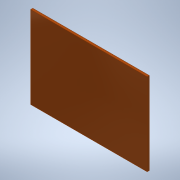
# Autodesk Inventor part: Yplate
Saved by Autodesk Inventor 2020 (Build 240168000, 168)
## iProperties
Created: 2019-06-14
Part Number: Yplate
Material: Phenolic Resin
Document SubType Name: Modeling
Designer: LillaHunden
Density: 1.38 g/cm^3
Appearance: Smooth - Light Orange
Author: LillaHunden
Autodesk Inventor part; units mm, degrees
ref_plane "YZ Plane" through (0, 0, 0) normal (1, 0, 0) x (0, 1, 0)
ref_plane "XZ Plane" through (0, 0, 0) normal (0, 1, 0) x (-1, 0, 0)
ref_plane "XY Plane" through (0, 0, 0) normal (0, 0, 1) x (1, 0, 0)
sketch "Sketch1" plane through (0, 0, 0) normal (0, 0, 1) x (1, 0, 0)
  line L0 (170, 120) -> (-170, 120)
  line L1 (-170, 120) -> (-170, -120)
  line L2 (-170, -120) -> (170, -120)
  line L3 (170, -120) -> (170, 120)
  line L4 (170, 120) -> (-170, -120) construction
  line L5 (-170, 120) -> (170, -120) construction
  point P0 (0, 0)
  dimension "d0" = 340
  dimension "d1" = 240
  constraints: 12 end point, 2 midpoint, 2 parallel, 1 horizontal, 1 perpendicular
  measures "d0" distance of L2.end L1.end
  measures "d1" distance of L1.end L0.end
extrude "Extrusion1" add sketch "Sketch1" along normal blind 6.35
body "Solid1"
